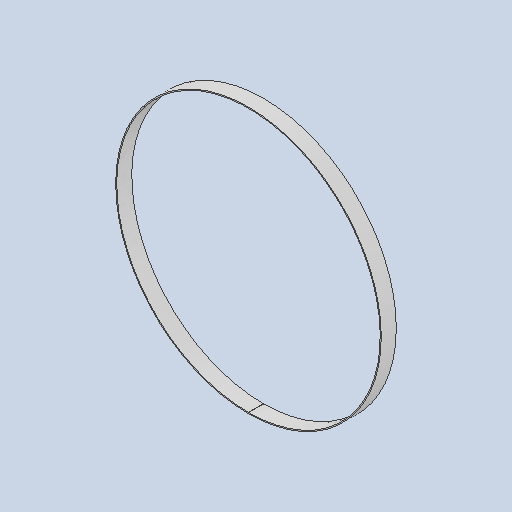
# Autodesk Inventor part: DMF2.0 01 46 Gear axis wheel 6
Saved by Autodesk Inventor 2025 (Build 290162010, 162A)
## iProperties
Created: 2024-04-30
Part Number: DMF2.0 01 46 Gear axis wheel 6
Material: Generic
Document SubType Name: Sheet Metal
Designer: admin
Stock Number: Барабан_Сектор_Усилителя
Density: 1 g/cm^3
Flat Pattern Width: 160.101 cm
Flat Pattern Length: 2.9 cm
Flat Pattern Area: 464.294 cm^2
Sheet Metal Rule: Default
Sheet Metal Width: 1601,013 mm
Sheet Metal Length: 29,000 mm
Sheet Metal Area: 46429,389 mm^2
Appearance: Default
Author: pokla
Autodesk Inventor part; units mm, degrees
note: some values were not read from the file. Chosen so that the rebuilt part matches the saved one: flange form of "Plate2".
ref_plane "YZ Plane" through (0, 0, 0) normal (1, 0, 0) x (0, 1, 0)
ref_plane "XZ Plane" through (0, 0, 0) normal (0, 1, 0) x (-1, 0, 0)
ref_plane "XY Plane" through (0, 0, 0) normal (0, 0, 1) x (1, 0, 0)
sketch "Sketch1" plane through (0, 0, 0) normal (0, 0, 1) x (1, 0, 0)
  arc A0 (0.2217, -253.9999) -> (-0.2217, -253.9999) centre (0, 0) ccw
  line L0 (0, 0) -> (-0.2217, -253.9999) construction
  line L1 (0, 0) -> (0, 241.44) construction
  line L2 (0, 0) -> (0.2217, -253.9999) construction
  arc A1 (-0.2217, -253.9999) -> (0.2217, -253.9999) centre (0, 0) ccw construction
  point P0 (-207.8461, 120)
  point P1 (207.8461, 120)
  dimension "d28" = 508
  dimension "d30" = 359.9
  measures "d28" diameter of A0
contour flange "Contour Flange1" sketch "Sketch1" thickness 2 bend radius 2 width 29 along (0, 0, 1) mid plane no both sides no wall seen from (0, 254, 0) lies toward (0, 1, 0) curves A0
bend "Bend1"
corner "Corner1"
equation "\"d28\" = Колесо_диам_3"
equation "\"d31\" = Thickness"
equation "\"d32\" = BendReliefWidth"
equation "\"d33\" = BendReliefDepth"
equation "\"d34\" = MinimumRemnant"
equation "\"d35\" = TransitionRadius"
equation "\"d37\" = BendRadius"
equation "\"d39\" = CornerReliefSize"
equation "\"d40\" = GapSize"
equation "\"d41\" = JacobiRadiusSize"
equation "\"BendRadius\" = Thickness"
equation "\"BendReliefWidth\" = Thickness"
equation "\"BendReliefDepth\" = 0.5 * Thickness"
equation "\"CornerReliefSize\" = 4 * Thickness"
equation "\"MinimumRemnant\" = 2 * Thickness"
equation "\"TransitionRadius\" = BendRadius"
equation "\"JacobiRadiusSize\" = BendRadius"
equation "\"GapSize\" = Thickness"
equation "\"Колесо_диам_3\" = 508"
equation "\"Thickness\" = 2"
body "Solid2"
